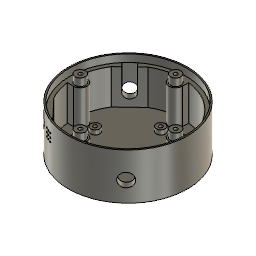
lamp pcb (Autodesk Fusion 360 archive; units mm, degrees)
design "WiFi_Controlled_Desk_Lamp_Base"
part number: 2026-05-20-15-05-35-264
Autodesk Fusion 360 part; units mm, degrees
note: some values were not read from the file. Chosen so that the rebuilt part matches the saved one: a direction; which face or edge a step refers to; which pieces of a blend or face edit are solid.
sketch "Sketch1" plane through (0, 0, 0) normal (0, 0, 1) x (1, 0, 0)
  circle A0 centre (0, 0) radius 40
  dimension "d1" = 80
  constraint coincident A0.centre origin
  measures "d1" diameter of A0
extrude "Extrude1" add sketch "Sketch1" along normal blind 31
shell "Shell1" thickness 2.5 removed faces 1 at (9.4847, -14.2223, 31)
sketch "Sketch2" plane through (0, 0, 31) normal (0, 0, 1) x (-1, 0, 0)
  circle A0 centre (0, 0) radius 37.5
  circle A1 centre (0, 0) radius 40
  circle A2 centre (0, 0) radius 39
  dimension "d5" = 78
  constraint concentric A0 A2
  measures "d5" diameter of A2
extrude "Extrude2" cut sketch "Sketch2" against normal blind 5 contours A0 | A2
sketch "Sketch3" plane through (0, 0, 31) normal (0, 0, 1) x (-1, 0, 0)
  circle A0 centre (0, 0) radius 39
  circle A1 centre (0, 0) radius 40
  circle A2 centre (-32, 0) radius 3.5
  circle A3 centre (-32, 0) radius 1.25
  dimension "d8" = 7
  dimension "d9" = 32
  dimension "d10" = 2.5
  constraint concentric A2 A3
  measures "d8" diameter of A2
  measures "d9" distance of A0.centre A2.centre
  measures "d10" diameter of A3
extrude "Extrude3" add sketch "Sketch3" against normal blind 29 contours A2
ref_plane "WorkPlane1" through (28.5, 0, 16.4689) normal (-1, 0, 0) x (0, -1, 0)
sketch "Sketch4" plane through (28.5, 0, 0) normal (-1, 0, 0) x (0, -1, 0)
  line L0 (3.5, 31) -> (-3.5, 31)
  line L1 (-3.5, 2.5) -> (3.5, 2.5)
  line L2 (3.5, 2.5) -> (-3.5, 2.5)
  line L3 (-3.5, 2.5) -> (-3.5, 26)
  line L4 (-3.5, 26) -> (3.5, 26)
  line L5 (3.5, 26) -> (3.5, 2.5)
  dimension "d14" = 23.5
  constraint perpendicular L2 L3
  constraint parallel L2 L4
  constraint parallel L3 L5
  constraint coincident L1.start L2.end
  constraint parallel L1 L2
  constraint coincident L1.end L2.start
  measures "d14" distance of L1.end L4.end
extrude "Extrude4" add sketch "Sketch4" against normal blind 5.5 from surface at -3.5
delete_face "DeleteFace1" 2 faces at (32, -0.4167, 18.1667) (32.8548, -0.5652, 26)
pattern_circular "C-Pattern1" count 4 over 360 about axis through (0, 0, 1.75) along (0, 0, 1) of "Extrude3", "Extrude4"
sketch "Sketch5" plane through (0, 0, 2.5) normal (0, 0, 1) x (-1, 0, 0)
  line L0 (-3.5, 32) -> (-3.5, 37.3363)
  line L1 (-37.3363, 3.5) -> (-32, 3.5)
  arc A0 (-32, -3.5) -> (-32, 3.5) centre (-32, 0) ccw
  line L2 (-32, -3.5) -> (-37.3363, -3.5)
  line L3 (-3.5, -37.3363) -> (-3.5, -32)
  arc A1 (3.5, -32) -> (-3.5, -32) centre (0, -32) ccw
  line L4 (3.5, -32) -> (3.5, -37.3363)
  line L5 (37.3363, -3.5) -> (32, -3.5)
  arc A2 (32, 3.5) -> (32, -3.5) centre (32, 0) ccw
  line L6 (32, 3.5) -> (37.3363, 3.5)
  line L7 (3.5, 37.3363) -> (3.5, 32)
  arc A3 (-3.5, 32) -> (3.5, 32) centre (0, 32) ccw
  circle A4 centre (22, 0) radius 3
  circle A5 centre (22, 0) radius 1.25
  arc A6 (-3.5, 37.3363) -> (-37.3363, 3.5) centre (0, 0) ccw
  arc A7 (-37.3363, -3.5) -> (-3.5, -37.3363) centre (0, 0) ccw
  arc A8 (3.5, -37.3363) -> (37.3363, -3.5) centre (0, 0) ccw
  arc A9 (37.3363, 3.5) -> (3.5, 37.3363) centre (0, 0) ccw
  dimension "d20" = 6
  dimension "d21" = 22
  dimension "d22" = 2.5
  constraint concentric A4 A5
  measures "d20" diameter of A4
  measures "d21" distance of A6.centre A4.centre
  measures "d22" diameter of A5
extrude "Extrude5" add sketch "Sketch5" along normal blind 3 contours A4
pattern_circular "C-Pattern2" count 4 over 360 about axis through (0, 0, 1.75) along (0, 0, 1) of "Extrude5"
delete_face "DeleteFace2" 2 faces at (0.4167, 32, 18.1667) (0.5652, 32.8548, 26)
delete_face "DeleteFace3" 2 faces at (-0.4167, -32, 18.1667) (0.0139, -32.8364, 26)
delete_face "DeleteFace4" 2 faces at (-32, 0.4167, 18.1667) (-32.6833, 0.3137, 26)
sketch "Sketch6" plane through (0, 0, 2.5) normal (0, 0, 1) x (-1, 0, 0)
  circle A0 centre (22, 0) radius 3
  line L0 (-3.5, 32) -> (-3.5, 37.3363)
  line L1 (-37.3363, 3.5) -> (-32, 3.5)
  arc A1 (-32, -3.5) -> (-32, 3.5) centre (-32, 0) ccw
  line L2 (-32, -3.5) -> (-37.3363, -3.5)
  line L3 (-3.5, -37.3363) -> (-3.5, -32)
  arc A2 (3.5, -32) -> (-3.5, -32) centre (0, -32) ccw
  line L4 (3.5, -32) -> (3.5, -37.3363)
  line L5 (37.3363, -3.5) -> (32, -3.5)
  arc A3 (32, 3.5) -> (32, -3.5) centre (32, 0) ccw
  line L6 (32, 3.5) -> (37.3363, 3.5)
  line L7 (3.5, 37.3363) -> (3.5, 32)
  arc A4 (-3.5, 32) -> (3.5, 32) centre (0, 32) ccw
  circle A5 centre (0, 22) radius 3
  circle A6 centre (-22, 0) radius 3
  circle A7 centre (0, -22) radius 3
  line L8 (18.7856, -32.4554) -> (31.6031, -20.1865)
  arc A8 (-3.5, 37.3363) -> (-37.3363, 3.5) centre (0, 0) ccw
  arc A9 (-37.3363, -3.5) -> (-3.5, -37.3363) centre (0, 0) ccw
  arc A10 (3.5, -37.3363) -> (37.3363, -3.5) centre (0, 0) ccw
  arc A11 (37.3363, 3.5) -> (3.5, 37.3363) centre (0, 0) ccw
  dimension "d27" = 17.743
  dimension "d28" = 16.046
  constraint coincident L8.start A8
  constraint coincident L8.end A8
  measures "d27" distance of L8.start L8.end
  measures "d28" distance of L4.end L8.start
extrude "Extrude6" add sketch "Sketch6" along normal blind 23.5 contours L8 A10
pattern_circular "C-Pattern3" count 3 over 180 about axis through (0, 0, 1.75) along (0, 0, 1) of "Extrude6"
sketch "Sketch7" plane through (25.1944, -26.3209, 0) normal (-0.691479, 0.722397, 0) x (-0.722397, -0.691479, 0)
  line L0 (8.8715, 26) -> (-8.8715, 26)
  circle A0 centre (0, 13.5) radius 4.5
  line L1 (-8.8715, 2.5) -> (8.8715, 2.5)
  line L2 (8.8715, 2.5) -> (8.8715, 26)
  line L3 (-8.8715, 26) -> (-8.8715, 2.5)
  dimension "d33" = 9
  dimension "d34" = 13.5
  measures "d33" diameter of A0
  measures "d34" distance of origin A0.centre
extrude "Extrude7" cut sketch "Sketch7" along normal through all and the other way through all contours A0
sketch "Sketch8" plane through (-25.1944, 26.3209, 0) normal (0.691479, -0.722397, 0) x (0.722397, 0.691479, 0)
  circle A0 centre (0, 13.5) radius 4.5
  line L0 (8.8715, 26) -> (-8.8715, 26)
  circle A1 centre (0, 11) radius 4.5
  line L1 (4.5, 11) -> (-4.5, 11)
  line L2 (-4.5, 11) -> (-4.5, 26)
  line L3 (4.5, 11) -> (4.5, 26)
  line L4 (-8.8715, 2.5) -> (8.8715, 2.5)
  line L5 (8.8715, 2.5) -> (8.8715, 26)
  line L6 (-8.8715, 26) -> (-8.8715, 2.5)
  point P0 (0, 11)
  dimension "d36" = 9
  dimension "d39" = 15
  constraint midpoint L1 P0
  constraint coincident P0 A1.centre
  constraint horizontal L1
  constraint coincident L0 L2.end
  constraint tangent A1 L2
  constraint perpendicular L0 L2
  constraint coincident L0 L3.end
  constraint tangent A0 L3
  constraint perpendicular L0 L3
  measures "d36" distance of L1.start L1.end
  measures "d39" distance of L1.start L3.end
delete_face "DeleteFace6" 1 faces at (-25.0585, 28.0859, 9.1975)
sketch "Sketch9" plane through (-25.1944, 26.3209, 0) normal (0.691479, -0.722397, 0) x (0.722397, 0.691479, 0)
  line L0 (-8.8715, 2.5) -> (8.8715, 2.5)
  line L1 (8.8715, 2.5) -> (8.8715, 26)
  line L2 (8.8715, 26) -> (-8.8715, 26)
  line L3 (-8.8715, 26) -> (-8.8715, 2.5)
  circle A0 centre (0, 11) radius 3.75
  line L4 (3.75, 11) -> (-3.75, 11)
  line L5 (-3.75, -4) -> (-3.75, 26)
  line L6 (3.75, -4) -> (3.75, 26)
  point P0 (0, 11)
  dimension "d40" = 7.5
  dimension "d41" = 11
  dimension "d42" = 7.5
  constraint midpoint L4 P0
  constraint coincident P0 A0.centre
  constraint horizontal L4
  constraint midpoint L4.end L5
  constraint coincident L2 L5.end
  constraint tangent A0 L5
  constraint perpendicular L2 L5
  constraint midpoint L4.start L6
  constraint coincident L2 L6.end
  constraint tangent A0 L6
  constraint perpendicular L2 L6
  measures "d40" diameter of A0
  measures "d41" distance of origin A0.centre
  measures "d42" distance of L4.start L4.end
extrude "Extrude9" cut sketch "Sketch9" against normal blind 2.6 contours L2 A0 L5 L6 | A0 L4 | A0 L4
extrude "Extrude10" cut sketch "Sketch9" against normal through all contours A0 L4 | A0 L4
sketch "Sketch10" plane through (-26.3209, -25.1944, 0) normal (0.722397, 0.691479, 0) x (-0.691479, 0.722397, 0)
  line L0 (-8.8715, 2.5) -> (8.8715, 2.5)
  line L1 (8.8715, 2.5) -> (8.8715, 26)
  line L2 (8.8715, 26) -> (-8.8715, 26)
  line L3 (-8.8715, 26) -> (-8.8715, 2.5)
  line L4 (-1.7405, 21.01) -> (-1.7405, 18.991)
  arc A0 (-1.7405, 18.991) -> (1.7405, 18.991) centre (0, 18.991) ccw
  line L5 (1.7405, 18.991) -> (1.7405, 21.01)
  arc A1 (1.7405, 21.01) -> (-1.7405, 21.01) centre (0, 21.01) ccw
  line L6 (0, 21.01) -> (0, 18.991) construction
  point P0 (0, 20.0005)
  dimension "d46" = 18.991
  dimension "d47" = 1.7405
  dimension "d48" = 5.5
  constraint tangent L4 A0
  constraint tangent A0 L5
  constraint parallel L4 L5
  constraint tangent L5 A1
  constraint tangent L4 A1
  constraint vertical L6
  constraint midpoint L6 P0
  constraint vertical origin P0
  measures "d46" distance of origin A0.centre
  measures "d47" radius of A1
extrude "Extrude11" cut sketch "Sketch10" against normal blind 0.698 contours L4 A0 L5 A1
extrude "Extrude12" cut 1 faces at (-26.424, -26.0961, 20.337) along direction (-0.722397, -0.691479, 0) through all draft 37
sketch "Sketch11" plane through (0, 0, 2.5) normal (0, 0, 1) x (-1, 0, 0)
  line L0 (-18.7856, 32.4554) -> (-31.6031, 20.1865)
  arc A0 (-31.6031, 20.1865) -> (-37.3363, 3.5) centre (0, 0) ccw
  line L1 (-37.3363, 3.5) -> (-32, 3.5)
  arc A1 (-32, -3.5) -> (-32, 3.5) centre (-32, 0) ccw
  line L2 (-32, -3.5) -> (-37.3363, -3.5)
  arc A2 (-37.3363, -3.5) -> (-3.5, -37.3363) centre (0, 0) ccw
  line L3 (-3.5, -37.3363) -> (-3.5, -32)
  arc A3 (3.5, -32) -> (-3.5, -32) centre (0, -32) ccw
  line L4 (3.5, -32) -> (3.5, -37.3363)
  arc A4 (3.5, -37.3363) -> (18.7856, -32.4554) centre (0, 0) ccw
  line L5 (18.7856, -32.4554) -> (31.6031, -20.1865)
  arc A5 (31.6031, -20.1865) -> (37.3363, -3.5) centre (0, 0) ccw
  line L6 (37.3363, -3.5) -> (32, -3.5)
  arc A6 (32, 3.5) -> (32, -3.5) centre (32, 0) ccw
  line L7 (32, 3.5) -> (37.3363, 3.5)
  arc A7 (37.3363, 3.5) -> (32.4554, 18.7856) centre (0, 0) ccw
  line L8 (32.4554, 18.7856) -> (20.1865, 31.6031)
  arc A8 (20.1865, 31.6031) -> (3.5, 37.3363) centre (0, 0) ccw
  line L9 (3.5, 37.3363) -> (3.5, 32)
  arc A9 (-3.5, 32) -> (3.5, 32) centre (0, 32) ccw
  line L10 (-3.5, 32) -> (-3.5, 37.3363)
  arc A10 (-3.5, 37.3363) -> (-18.7856, 32.4554) centre (0, 0) ccw
  circle A11 centre (22, 0) radius 3
  circle A12 centre (0, 22) radius 3
  circle A13 centre (-22, 0) radius 3
  circle A14 centre (0, -22) radius 3
  arc A15 (-4.5, 32) -> (4.5, 32) centre (0, 32) ccw
  line L11 (4.5, 36.2215) -> (4.5, 32)
  arc A16 (19.5476, 30.8244) -> (4.5, 36.2215) centre (0, 0) ccw
  line L12 (31.6494, 18.1814) -> (19.5476, 30.8244)
  arc A17 (36.2215, 4.5) -> (31.6494, 18.1814) centre (0, 0) ccw
  line L13 (32, 4.5) -> (36.2215, 4.5)
  arc A18 (32, 4.5) -> (32, -4.5) centre (32, 0) ccw
  line L14 (36.2215, -4.5) -> (32, -4.5)
  arc A19 (30.8244, -19.5476) -> (36.2215, -4.5) centre (0, 0) ccw
  line L15 (18.1814, -31.6494) -> (30.8244, -19.5476)
  arc A20 (4.5, -36.2215) -> (18.1814, -31.6494) centre (0, 0) ccw
  line L16 (4.5, -32) -> (4.5, -36.2215)
  arc A21 (4.5, -32) -> (-4.5, -32) centre (0, -32) ccw
  line L17 (-4.5, -36.2215) -> (-4.5, -32)
  arc A22 (-36.2215, -4.5) -> (-4.5, -36.2215) centre (0, 0) ccw
  line L18 (-32, -4.5) -> (-36.2215, -4.5)
  arc A23 (-32, -4.5) -> (-32, 4.5) centre (-32, 0) ccw
  line L19 (-36.2215, 4.5) -> (-32, 4.5)
  arc A24 (-30.8244, 19.5476) -> (-36.2215, 4.5) centre (0, 0) ccw
  line L20 (-18.1814, 31.6494) -> (-30.8244, 19.5476)
  arc A25 (-4.5, 36.2215) -> (-18.1814, 31.6494) centre (0, 0) ccw
  line L21 (-4.5, 32) -> (-4.5, 36.2215)
  dimension "d52" = -1
extrude "Extrude13" add sketch "Sketch11" along normal blind 23.5 contours L0 A0 L1 A1 L2 A2 L3 A3 L4 A4 L5 A5 L6 A6 L7 A7 L8 A8 L9 A9 L10 A10
delete_face "DeleteFace7" 1 faces at (24.5188, -26.9676, 14.6727)
delete_face "DeleteFace8" 1 faces at (-24.2914, 27.1853, 16)
delete_face "DeleteFace9" 1 faces at (-26.7221, -24.7753, 19.664)
sketch "Sketch12" plane through (0, 0, 26) normal (0, 0, 1) x (-1, 0, 0)
  line L0 (24.1337, -30.636) -> (21.7939, -28.1916)
  line L1 (21.7939, -28.1916) -> (18.1814, -31.6494)
  arc A0 (4.5, -36.2215) -> (18.1814, -31.6494) centre (0, 0) ccw
  line L2 (4.5, -36.2215) -> (4.5, -32)
  arc A1 (4.5, -32) -> (-4.5, -32) centre (0, -32) ccw
  line L3 (-4.5, -32) -> (-4.5, -36.2215)
  arc A2 (-36.2215, -4.5) -> (-4.5, -36.2215) centre (0, 0) ccw
  line L4 (-36.2215, -4.5) -> (-32, -4.5)
  arc A3 (-32, -4.5) -> (-32, 4.5) centre (-32, 0) ccw
  line L5 (-32, 4.5) -> (-36.2215, 4.5)
  arc A4 (-30.8244, 19.5476) -> (-36.2215, 4.5) centre (0, 0) ccw
  line L6 (-30.8244, 19.5476) -> (-18.1814, 31.6494)
  arc A5 (-4.5, 36.2215) -> (-18.1814, 31.6494) centre (0, 0) ccw
  line L7 (-4.5, 36.2215) -> (-4.5, 32)
  arc A6 (-4.5, 32) -> (4.5, 32) centre (0, 32) ccw
  line L8 (4.5, 32) -> (4.5, 36.2215)
  arc A7 (19.5476, 30.8244) -> (4.5, 36.2215) centre (0, 0) ccw
  line L9 (19.5476, 30.8244) -> (31.6494, 18.1814)
  arc A8 (36.2215, 4.5) -> (31.6494, 18.1814) centre (0, 0) ccw
  line L10 (36.2215, 4.5) -> (32, 4.5)
  arc A9 (32, 4.5) -> (32, -4.5) centre (32, 0) ccw
  line L11 (32, -4.5) -> (36.2215, -4.5)
  arc A10 (30.8244, -19.5476) -> (36.2215, -4.5) centre (0, 0) ccw
  line L12 (30.8244, -19.5476) -> (27.2119, -23.0055)
  line L13 (27.2119, -23.0055) -> (29.5517, -25.4499)
  arc A11 (29.5517, -25.4499) -> (24.1337, -30.636) centre (0, 0) ccw
  circle A12 centre (0, -32) radius 3.5
  circle A13 centre (-32, 0) radius 3.5
  circle A14 centre (32, 0) radius 3.5
  circle A15 centre (0, 32) radius 3.5
  line L14 (21.1305, 31.8051) -> (11.6117, 36.2372)
  line L15 (21.1305, 31.8051) -> (20.3053, 30.0328)
  line L16 (11.6117, 36.2372) -> (10.9511, 34.8184)
  dimension "d55" = 10.5
  dimension "d56" = 17.212
  dimension "d57" = 1.565
  dimension "d58" = 1.955
  constraint coincident L9 L15.end
  constraint perpendicular L14 L15
  constraint coincident A7 L16.end
  constraint perpendicular L14 L16
  measures "d55" distance of L14.start L14.end
  measures "d56" distance of L9.end L14.start
  measures "d57" distance of L14.end L16.end
  measures "d58" distance of L14.start L15.end
extrude "Extrude14" cut sketch "Sketch12" against normal blind 5.8 contours A7 L9 L14 L15 L16
ref_plane "WorkPlane2" through (-20.3053, -30.0328, 26) normal (0.364607, 0.931162, 0) x (-0.931162, 0.364607, 0)
sketch "Sketch13" plane through (-12.8957, -32.9341, 0) normal (0.364607, 0.931162, 0) x (-0.931162, 0.364607, 0)
  line L0 (7.9573, 26) -> (7.9573, 20.2)
  line L1 (-2.4978, 20.2) -> (-2.4978, 26)
  line L2 (6.9632, 20.2) -> (-2.4978, 20.2)
  line L3 (7.9573, 20.2) -> (6.9632, 20.2)
  arc A0 (-2.4978, 20.2) -> (7.9573, 20.2) centre (2.7298, 20.2) ccw
  constraint tangent L0 A0
extrude "Extrude15" cut sketch "Sketch13" along normal up to surface end surface through (-21.1305, -31.8051, 26) normal (0.422101, 0.906549, 0) offset 0
sketch "Sketch14" plane through (-15.9352, -34.2241, 0) normal (0.422101, 0.906549, 0) x (-0.906549, 0.422101, 0)
  line L0 (5.7308, 26) -> (-4.7692, 26)
  line L1 (-4.7692, 26) -> (-4.7692, 20.2)
  line L2 (-4.7692, 20.2) -> (-4.8672, 20.2)
  ellipse E0 centre (0.3706, 20.2) end of major axis (-4.8672, 20.2) minor radius 5.2275 (-4.8672, 20.2) -> (5.6084, 20.2) ccw
  line L3 (5.6084, 20.2) -> (5.7308, 20.2)
  line L4 (5.7308, 20.2) -> (5.7308, 26)
  circle A0 centre (2.8298, 23.4) radius 0.6
  circle A1 centre (0.5118, 23.4) radius 0.6
  circle A2 centre (-1.8062, 23.4) radius 0.6
  circle A3 centre (2.8298, 20.9) radius 0.6
  circle A4 centre (0.5118, 20.9) radius 0.6
  circle A5 centre (-1.8062, 20.9) radius 0.6
  circle A6 centre (2.8298, 18.4) radius 0.6
  circle A7 centre (0.5118, 18.4) radius 0.6
  circle A8 centre (-1.8062, 18.4) radius 0.6
  dimension "d63" = 1.2
  dimension "d64" = 2.6
  dimension "d65" = 2.901
  dimension "d68" = -4.636
  dimension "d69" = 0
  dimension "d72" = 0
  dimension "d73" = -5
  measures "d63" diameter of A0
  measures "d64" distance of L0 A0.centre
  measures "d65" distance of L4 A0.centre
extrude "Extrude16" cut sketch "Sketch14" against normal through all contours A0 | A1 | A2 | A3 | A4 | A5 | A6 | A7 | A8
equation "d29 = 22.5 mm + 1 mm"
equation "d41 = 7.25 mm + 3.75 mm"
equation "d47 = ( 3.481 / 2 ) * 1 mm"
equation "d68 = ( -2.318 * 2 ) * 1 mm"
